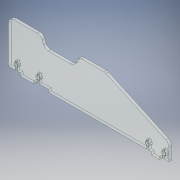
# Autodesk Inventor part: Soporte_Ambu_Der
Saved by Autodesk Inventor 2019 (Build 230136000, 136)
## iProperties
Created: 2020-04-04
Part Number: Soporte_Ambu_Der
Material: Generic
Document SubType Name: Modeling
Designer: Jurgen
Density: 1 g/cm^3
Appearance: Clear
Mass: 104.22 g
Surface Area: 463.388 cm^2
Volume: 104.22 cm^3
Author: Jurgen
Autodesk Inventor part; units mm, degrees
ref_plane "YZ Plane" through (0, 0, 0) normal (1, 0, 0) x (0, 1, 0)
ref_plane "XZ Plane" through (0, 0, 0) normal (0, 1, 0) x (-1, 0, 0)
ref_plane "XY Plane" through (0, 0, 0) normal (0, 0, 1) x (1, 0, 0)
sketch "Sketch1" plane through (0, 0, 0) normal (0, 0, 1) x (1, 0, 0)
  circle A0 centre (0, 0) radius 63.5 construction
  line L0 (0, 0) -> (-110.5, 0) construction
  line L1 (-110.5, 0) -> (-110.5, -80) construction
  line L2 (-110.5, -80) -> (-35.5, -80) construction
  line L3 (0, 0) -> (189.5, 0) construction
  line L4 (189.5, 0) -> (189.5, -85) construction
  line L5 (189.5, -85) -> (134.5, -85) construction
  line L6 (-93, -80) -> (-53, -80) construction
  line L7 (-53, -80) -> (-53, -85) construction
  line L8 (-53, -85) -> (-93, -85) construction
  line L9 (-93, -85) -> (-93, -80) construction
  line L10 (147, -85) -> (177, -85) construction
  line L11 (177, -85) -> (177, -90) construction
  line L12 (177, -90) -> (147, -90) construction
  line L13 (147, -90) -> (147, -85) construction
  circle A1 centre (0, 0) radius 18.5 construction
  line L14 (-35.5, -80) -> (134.5, -85) construction
  line L15 (0, 0) -> (0, -63.5) construction
  line L16 (-20.0131, 0) -> (0, -48.5) construction
  line L17 (20.0131, 0) -> (0, -48.5) construction
  line L18 (-53, -80) -> (-53, -85)
  line L19 (-53, -85) -> (-93, -85)
  line L20 (-93, -85) -> (-93, -80)
  line L21 (-93, -80) -> (-110.5, -80)
  line L22 (-110.5, -80) -> (-110.5, 0)
  line L23 (-110.5, 0) -> (-20.0131, 0) construction
  line L24 (-20.0131, 0) -> (0, -48.5) construction
  line L25 (0, -48.5) -> (20.0131, 0) construction
  line L26 (20.0131, 0) -> (189.5, 0) construction
  line L27 (189.5, 0) -> (189.5, -85) construction
  line L28 (189.5, -85) -> (177, -85)
  line L29 (177, -85) -> (177, -90)
  line L30 (177, -90) -> (147, -90)
  line L31 (147, -90) -> (147, -85)
  line L32 (147, -85) -> (79.5, -85)
  line L33 (-53, -80) -> (-35.5, -80)
  line L34 (-35.5, -80) -> (-35.5, -85)
  line L35 (-35.5, -85) -> (79.5, -85)
  line L36 (20.0131, 0) -> (70.0131, 0)
  line L37 (70.0131, 0) -> (189.5, -55)
  line L38 (189.5, -55) -> (189.5, -85)
  line L39 (0, -48.5) -> (-30, -48.5) construction
  line L40 (-30, -48.5) -> (-50.0131, 0) construction
  line L41 (12.3793, -18.5) -> (-42.3793, -18.5) construction
  line L42 (-110.5, 0) -> (-50.0131, 0)
  line L43 (-50.0131, 0) -> (-42.3793, -18.5)
  line L44 (-42.3793, -18.5) -> (12.3793, -18.5)
  line L45 (12.3793, -18.5) -> (20.0131, 0)
  dimension "d0" = 127
  dimension "d1" = 110.5
  dimension "d2" = 80
  dimension "d3" = 75
  dimension "d4" = 189.5
  dimension "d5" = 85
  dimension "d6" = 55
  dimension "d7" = 40
  dimension "d8" = 5
  dimension "d9" = 17.5
  dimension "d10" = 30
  dimension "d11" = 5
  dimension "d12" = 42.5
  dimension "d13" = 37
  dimension "d14" = 15
  dimension "d18" = 50
  dimension "d19" = 30
  dimension "d59" = 30
  constraints: 92 end point, 15 perpendicular, 10 point on line, 7 parallel, 6 horizontal, 5 vertical, 4 collinear, 3 tangent, 2 coincident, 1 centre point, 1 vertical alignment, 2 other
  measures "d1" distance of L0.start L0.end
  measures "d2" distance of L0.end L1.end
  measures "d3" distance of L1.end L2.end
  measures "d4" distance of L0.start L3.end
  measures "d5" distance of L3.end L4.end
  measures "d6" distance of L4.end L5.end
  measures "d7" distance of L7.end L8.end
  measures "d8" distance of L6.end L7.end
  measures "d9" distance from line of L2.end L7
  measures "d10" distance of L11.end L12.end
  measures "d11" distance of L10.end L11.end
  measures "d12" distance between parallel lines of L4 L13
  measures "d13" diameter of A1
  measures "d14" distance of L16.end L15.end
  measures "d18" distance of L17.start L36.end
  measures "d19" distance of L4.end L37.end
  measures "d59" distance of L16.end L39.end
extrude "Extrusion1" add sketch "Sketch1" along normal blind 5
fillet "Fillet1" radius 10 4 edges at (-110.5, 0, 2.5) (20.0131, 0, 2.5) (70.0131, 0, 2.5) (189.5, -55, 2.5)
sketch "Sketch2" plane through (0, 0, 5) normal (0, 0, 1) x (1, 0, 0)
  circle A0 centre (0, 0) radius 63.5 construction
  line L0 (0, 0) -> (-110.5, 0) construction
  line L1 (-110.5, 0) -> (-110.5, -80) construction
  line L2 (0, 0) -> (189.5, 0) construction
  line L3 (189.5, 0) -> (189.5, -85) construction
  line L4 (-88, -80) -> (-63, -80) construction
  line L5 (-63, -80) -> (-63, -85) construction
  line L6 (-63, -85) -> (-88, -85) construction
  line L7 (-88, -85) -> (-88, -80) construction
  line L8 (157, -85) -> (172, -85) construction
  line L9 (172, -85) -> (172, -90) construction
  line L10 (172, -90) -> (157, -90) construction
  line L11 (157, -90) -> (157, -85) construction
  circle A1 centre (0, 0) radius 33.5 construction
  line L12 (-35.5, -80) -> (134.5, -85) construction
  line L13 (0, 0) -> (0, -63.5) construction
  line L14 (-40.8636, 0) -> (0, -58.5) construction
  line L15 (40.8636, 0) -> (0, -58.5) construction
  line L16 (-63, -80) -> (-63, -85) construction
  line L17 (-63, -85) -> (-88, -85) construction
  line L18 (-88, -85) -> (-88, -80) construction
  line L19 (-110.5, -80) -> (-110.5, 0) construction
  line L20 (-110.5, 0) -> (-40.8636, 0) construction
  line L21 (-40.8636, 0) -> (0, -58.5) construction
  line L22 (0, -58.5) -> (40.8636, 0) construction
  line L23 (40.8636, 0) -> (189.5, 0) construction
  line L24 (189.5, 0) -> (189.5, -85) construction
  line L25 (172, -85) -> (172, -90) construction
  line L26 (172, -90) -> (157, -90) construction
  line L27 (157, -90) -> (157, -85) construction
  line L28 (-35.5, -80) -> (-35.5, -85) construction
  line L29 (-35.5, -85) -> (94.5, -85) construction
  line L30 (40.8636, 0) -> (70.8636, 0) construction
  line L31 (70.8636, 0) -> (189.5, -55) construction
  line L32 (189.5, -55) -> (189.5, -85) construction
  line L33 (151, -85) -> (145, -85) construction
  line L34 (172, -85) -> (178, -85) construction
  line L35 (151, -85) -> (149, -85) construction
  line L36 (147, -85) -> (147, -70) construction
  line L37 (147, -70) -> (151, -70) construction
  line L38 (151, -70) -> (151, -85) construction
  line L39 (149, -70) -> (149, -85) construction
  line L40 (145, -78) -> (153, -78) construction
  line L41 (153, -78) -> (153, -74) construction
  line L42 (153, -74) -> (145, -74) construction
  line L43 (145, -74) -> (145, -78) construction
  line L44 (145, -78) -> (153, -74) construction
  line L45 (153, -78) -> (145, -74) construction
  line L46 (180, -85) -> (182, -85) construction
  line L47 (182, -85) -> (182, -70) construction
  line L48 (182, -70) -> (178, -70) construction
  line L49 (178, -70) -> (178, -85) construction
  line L50 (180, -70) -> (180, -85) construction
  line L51 (184, -78) -> (176, -78) construction
  line L52 (176, -78) -> (176, -74) construction
  line L53 (176, -74) -> (184, -74) construction
  line L54 (184, -74) -> (184, -78) construction
  line L55 (184, -78) -> (176, -74) construction
  line L56 (176, -78) -> (184, -74) construction
  line L57 (147, -85) -> (147, -78) construction
  line L58 (147, -85) -> (147, -78) construction
  line L59 (147, -78) -> (145, -78) construction
  line L60 (145, -78) -> (145, -74) construction
  line L61 (145, -74) -> (147, -74) construction
  line L62 (147, -74) -> (147, -70) construction
  line L63 (147, -70) -> (151, -70) construction
  line L64 (151, -70) -> (151, -74) construction
  line L65 (151, -74) -> (153, -74) construction
  line L66 (153, -74) -> (153, -78) construction
  line L67 (153, -78) -> (151, -78) construction
  line L68 (151, -78) -> (151, -85) construction
  line L69 (147, -85) -> (134.5, -85) construction
  line L70 (157, -85) -> (151, -85) construction
  line L71 (147, -85) -> (94.5, -85) construction
  line L72 (178, -85) -> (178, -78) construction
  line L73 (178, -78) -> (176, -78) construction
  line L74 (176, -78) -> (176, -74) construction
  line L75 (176, -74) -> (178, -74) construction
  line L76 (178, -74) -> (178, -70) construction
  line L77 (178, -70) -> (182, -70) construction
  line L78 (182, -70) -> (182, -74) construction
  line L79 (182, -74) -> (184, -74) construction
  line L80 (184, -74) -> (184, -78) construction
  line L81 (184, -78) -> (182, -78) construction
  line L82 (182, -78) -> (182, -85) construction
  line L83 (189.5, -85) -> (180, -85) construction
  line L84 (178, -85) -> (149, -85) construction
  line L85 (189.5, -85) -> (182, -85) construction
  line L86 (178, -85) -> (172, -85) construction
  line L87 (-98, -80) -> (-98, -65) construction
  line L88 (-98, -65) -> (-94, -65) construction
  line L89 (-94, -65) -> (-94, -80) construction
  line L90 (-55, -80) -> (-53, -80) construction
  line L91 (-53, -80) -> (-53, -65) construction
  line L92 (-53, -65) -> (-57, -65) construction
  line L93 (-57, -65) -> (-57, -80) construction
  line L94 (-96, -65) -> (-96, -80) construction
  line L95 (-55, -65) -> (-55, -80) construction
  line L96 (-100, -73) -> (-92, -73) construction
  line L97 (-92, -73) -> (-92, -69) construction
  line L98 (-92, -69) -> (-100, -69) construction
  line L99 (-100, -69) -> (-100, -73) construction
  line L100 (-100, -73) -> (-92, -69) construction
  line L101 (-92, -73) -> (-100, -69) construction
  line L102 (-51, -73) -> (-59, -73) construction
  line L103 (-59, -73) -> (-59, -69) construction
  line L104 (-59, -69) -> (-51, -69) construction
  line L105 (-51, -69) -> (-51, -73) construction
  line L106 (-51, -73) -> (-59, -69) construction
  line L107 (-59, -73) -> (-51, -69) construction
  line L108 (-98, -80) -> (-98, -73) construction
  line L109 (-98, -73) -> (-100, -73) construction
  line L110 (-100, -73) -> (-100, -69) construction
  line L111 (-100, -69) -> (-98, -69) construction
  line L112 (-98, -69) -> (-98, -65) construction
  line L113 (-98, -65) -> (-94, -65) construction
  line L114 (-94, -65) -> (-94, -69) construction
  line L115 (-94, -69) -> (-92, -69) construction
  line L116 (-92, -69) -> (-92, -73) construction
  line L117 (-92, -73) -> (-94, -73) construction
  line L118 (-94, -73) -> (-94, -80) construction
  line L119 (-88, -80) -> (-94, -80) construction
  line L120 (-98, -80) -> (-110.5, -80) construction
  line L121 (-57, -80) -> (-57, -73) construction
  line L122 (-57, -73) -> (-59, -73) construction
  line L123 (-59, -73) -> (-59, -69) construction
  line L124 (-59, -69) -> (-57, -69) construction
  line L125 (-57, -69) -> (-57, -65) construction
  line L126 (-57, -65) -> (-53, -65) construction
  line L127 (-53, -65) -> (-53, -69) construction
  line L128 (-53, -69) -> (-51, -69) construction
  line L129 (-51, -69) -> (-51, -73) construction
  line L130 (-51, -73) -> (-53, -73) construction
  line L131 (-53, -73) -> (-53, -80) construction
  line L132 (-110.5, -80) -> (-57, -80) construction
  line L133 (-55, -80) -> (-35.5, -80) construction
  line L134 (-63, -80) -> (-57, -80) construction
  line L135 (-53, -80) -> (-35.5, -80) construction
  line L136 (-88, -85) -> (-94, -85)
  line L137 (-94, -85) -> (-94, -80)
  line L138 (-94, -80) -> (-88, -80)
  line L139 (-88, -80) -> (-88, -85)
  line L140 (-94, -80) -> (-98, -80)
  line L141 (-98, -80) -> (-98, -73)
  line L142 (-98, -73) -> (-100, -73)
  line L143 (-100, -69) -> (-100, -73)
  line L144 (-100, -69) -> (-98, -69)
  line L145 (-98, -69) -> (-98, -65)
  line L146 (-98, -65) -> (-94, -65)
  line L147 (-94, -65) -> (-94, -69)
  line L148 (-94, -69) -> (-92, -69)
  line L149 (-92, -69) -> (-92, -73)
  line L150 (-92, -73) -> (-94, -73)
  line L151 (-94, -73) -> (-94, -80)
  line L152 (-110.5, -80) -> (-93, -80) projected
  line L153 (-63, -80) -> (-63, -85)
  line L154 (-63, -85) -> (-53, -85)
  line L155 (-53, -85) -> (-53, -73)
  line L156 (-53, -73) -> (-51, -73)
  line L157 (-51, -73) -> (-51, -69)
  line L158 (-51, -69) -> (-53, -69)
  line L159 (-53, -69) -> (-53, -65)
  line L160 (-53, -65) -> (-57, -65)
  line L161 (-57, -65) -> (-57, -69)
  line L162 (-57, -69) -> (-59, -69)
  line L163 (-59, -69) -> (-59, -73)
  line L164 (-59, -73) -> (-57, -73)
  line L165 (-57, -73) -> (-57, -80)
  line L166 (-57, -80) -> (-63, -80)
  line L167 (157, -85) -> (157, -90)
  line L168 (157, -90) -> (147, -90)
  line L169 (147, -90) -> (147, -78)
  line L170 (147, -78) -> (145, -78)
  line L171 (145, -78) -> (145, -74)
  line L172 (145, -74) -> (147, -74)
  line L173 (147, -74) -> (147, -70)
  line L174 (147, -70) -> (151, -70)
  line L175 (151, -70) -> (151, -74)
  line L176 (151, -74) -> (153, -74)
  line L177 (153, -74) -> (153, -78)
  line L178 (153, -78) -> (151, -78)
  line L179 (151, -78) -> (151, -85)
  line L180 (151, -85) -> (157, -85)
  line L181 (147, -90) -> (177, -90) projected
  line L182 (172, -90) -> (177, -90)
  line L183 (177, -90) -> (177, -85)
  line L184 (177, -85) -> (172, -85)
  line L185 (172, -85) -> (172, -90)
  line L186 (178, -85) -> (178, -78)
  line L187 (178, -78) -> (176, -78)
  line L188 (176, -78) -> (176, -74)
  line L189 (176, -74) -> (178, -74)
  line L190 (178, -74) -> (178, -70)
  line L191 (178, -70) -> (182, -70)
  line L192 (182, -70) -> (182, -74)
  line L193 (182, -74) -> (184, -74)
  line L194 (184, -74) -> (184, -78)
  line L195 (184, -78) -> (182, -78)
  line L196 (182, -78) -> (182, -85)
  line L197 (182, -85) -> (178, -85)
  point P0 (149, -76)
  point P1 (180, -76)
  point P2 (-96, -71)
  point P3 (-55, -71)
  dimension "d20" = 127
  dimension "d21" = 110.5
  dimension "d22" = 80
  dimension "d23" = 75
  dimension "d24" = 189.5
  dimension "d25" = 85
  dimension "d26" = 55
  dimension "d27" = 25
  dimension "d28" = 5
  dimension "d29" = 27.5
  dimension "d30" = 15
  dimension "d31" = 5
  dimension "d32" = 67
  dimension "d33" = 5
  dimension "d34" = 30
  dimension "d35" = 30
  dimension "d36" = 17.5
  dimension "d37" = 6
  dimension "d38" = 4
  dimension "d39" = 15
  dimension "d40" = 8
  dimension "d41" = 4
  dimension "d42" = 4
  dimension "d43" = 8
  dimension "d44" = 6
  dimension "d45" = 4
  dimension "d46" = 15
  dimension "d47" = 6
  dimension "d48" = 4
  dimension "d49" = 15
  dimension "d50" = 6
  dimension "d51" = 8
  dimension "d52" = 4
  dimension "d53" = 8
  dimension "d54" = 7
  dimension "d55" = 7
  dimension "d56" = 12.5
  constraints: 393 end point, 81 perpendicular, 46 point on line, 29 parallel, 25 collinear, 18 horizontal, 12 midpoint, 7 vertical, 2 coincident, 2 tangent, 1 centre point, 1 vertical alignment, 2 other
  measures "d21" distance of L0.start L0.end
  measures "d22" distance of L0.end L1.end
  measures "d23" distance of L1.end L12.start
  measures "d24" distance of L0.start L2.end
  measures "d25" distance of L2.end L3.end
  measures "d26" distance of L3.end L12.end
  measures "d27" distance of L5.end L6.end
  measures "d28" distance of L4.end L5.end
  measures "d29" distance from line of L12.start L5
  measures "d30" distance of L9.end L10.end
  measures "d31" distance of L8.end L9.end
  measures "d32" diameter of A1
  measures "d33" distance of L14.end L13.end
  measures "d34" distance of L30.end L15.start
  measures "d35" distance of L3.end L31.end
  measures "d36" distance between parallel lines of L32 L9
  measures "d37" distance of L34.end L8.end
  measures "d38" distance of L36.end L37.end
  measures "d39" distance of L36.start L36.end
  measures "d40" distance of L42.end L41.end
  measures "d41" distance of L41.end L40.end
  measures "d42" distance of L48.end L47.end
  measures "d43" distance of L52.end L53.end
  measures "d44" distance between parallel lines of L11 L38
  measures "d45" distance of L87.end L88.end
  measures "d46" distance of L87.start L87.end
  measures "d47" distance between parallel lines of L7 L89
  measures "d48" distance of L92.end L91.end
  measures "d49" distance of L91.end L90.end
  measures "d50" distance between parallel lines of L5 L93
  measures "d51" distance of L98.end L97.end
  measures "d52" distance of L97.end L96.end
  measures "d53" distance of L103.end L104.end
  measures "d54" distance between parallel lines of L119 L117
  measures "d55" distance between parallel lines of L132 L102
  measures "d56" distance between parallel lines of L19 L108
extrude "Extrusion2" cut sketch "Sketch2" against normal blind 5
fillet "Fillet2" radius 10 3 edges at (-50.0131, 0, 2.5) (-42.3793, -18.5, 2.5) (12.3793, -18.5, 2.5)
body "Solid1"
